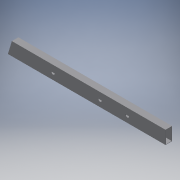
# Autodesk Inventor part: Aluminum Channel Arm
Saved by Autodesk Inventor 2019 (Build 230136000, 136)
## iProperties
Created: 2019-01-26
Part Number: Aluminum Channel Arm
Material: Generic
Document SubType Name: Modeling
Designer: josh
Density: 1 g/cm^3
Appearance: Default
Mass: 112.762 g
Surface Area: 1783.03 cm^2
Volume: 112.762 cm^3
Author: josh
Autodesk Inventor part; units mm, degrees
ref_plane "YZ Plane" through (0, 0, 0) normal (1, 0, 0) x (0, 1, 0)
ref_plane "XZ Plane" through (0, 0, 0) normal (0, 1, 0) x (-1, 0, 0)
ref_plane "XY Plane" through (0, 0, 0) normal (0, 0, 1) x (1, 0, 0)
sketch "Sketch1" plane through (0, 0, 0) normal (1, 0, 0) x (0, 1, 0)
  line L0 (0, 0) -> (50.8, 0)
  line L1 (50.8, 0) -> (50.8, -25.4)
  line L2 (50.8, -25.4) -> (0, -25.4)
  line L3 (0, -25.4) -> (0, 0)
  line L4 (49.53, -24.13) -> (49.53, -1.27)
  line L5 (49.53, -1.27) -> (1.27, -1.27)
  line L6 (1.27, -1.27) -> (1.27, -24.13)
  line L7 (1.27, -24.13) -> (49.53, -24.13)
  dimension "d0" = 50.8
  dimension "d1" = 25.4
  dimension "d2" = 1.27
  constraints: 16 end point, 4 parallel, 2 perpendicular, 1 horizontal, 3 other
  measures "d0" distance of L1.end L2.end
  measures "d1" distance of L0.end L1.end
  measures "d2" distance between parallel lines of L1 L4
extrude "Extrusion1" add sketch "Sketch1" along normal blind 609.6
sketch "Sketch2" plane through (0, 0, -25.4) normal (0, 0, -1) x (-1, 0, 0)
  circle A0 centre (-174.2245, 25.4) radius 7.3323
  circle A1 centre (-355.8783, 25.3733) radius 7.3323
  line L0 (-461.8402, 31.7005) -> (-458.3441, 31.8328) projected
  arc A2 (-458.0874, 31.6973) -> (-458.3441, 31.8328) centre (-461.6, 25.355) ccw projected
  arc A3 (-454.3512, 25.4841) -> (-454.3621, 25.7742) centre (-461.6, 25.355) ccw projected
  arc A4 (-457.8637, 19.1419) -> (-457.618, 19.2964) centre (-461.6, 25.355) ccw projected
  arc A5 (-465.3363, 31.5681) -> (-465.582, 31.4136) centre (-461.6, 25.355) ccw projected
  arc A6 (-468.8488, 25.2259) -> (-468.8379, 24.9358) centre (-461.6, 25.355) ccw projected
  arc A7 (-465.1126, 19.0127) -> (-464.8559, 18.8772) centre (-461.6, 25.355) ccw projected
  arc A8 (-457.8637, 19.1419) -> (-457.618, 19.2964) centre (-461.6, 25.355) ccw projected
  circle A9 centre (-461.8402, 25.355) radius 7.3767
  line L1 (0, 0) -> (-15.2407, 50.8)
  line L2 (0, 50.8) -> (-609.6, 50.8) projected
  line L3 (0, 0) -> (53.037, 0) construction
  line L4 (0, 0) -> (0, 50.8)
  line L5 (-15.2407, 50.8) -> (0, 50.8)
  dimension "d7" = 14.6647
  dimension "d9" = 106.7
  constraints: 8 end point, 2 centre point, 2 horizontal, 1 equal length, 1 equal radius, 1 point on line, 1 vertical, 3 other
  measures "d7" diameter of A0
  measures "d9" angle of L3 L1
extrude "Extrusion2" cut sketch "Sketch2" against normal through all
body "Solid1"
